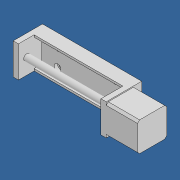
# Autodesk Inventor part: Linear_Unit_A
Saved by Autodesk Inventor 2020 (Build 240168000, 168)
## iProperties
Created: 2021-07-13
Part Number: Linear_Unit_A
Material: 一般
Document SubType Name: Modeling
Designer: ken113
Density: 1 g/cm^3
Appearance: 既定
Author: ken113
Autodesk Inventor part; units mm, degrees
ref_plane "YZ Plane" through (0, 0, 0) normal (1, 0, 0) x (0, 1, 0)
ref_plane "XZ Plane" through (0, 0, 0) normal (0, 1, 0) x (-1, 0, 0)
ref_plane "XY Plane" through (0, 0, 0) normal (0, 0, 1) x (1, 0, 0)
sketch "スケッチ1" plane through (0, 0, 0) normal (0, 0, 1) x (1, 0, 0)
  line L0 (62.5, -15) -> (-62.5, -15)
  line L1 (-62.5, -15) -> (-62.5, 15)
  line L2 (-62.5, 15) -> (62.5, 15)
  line L3 (62.5, 15) -> (62.5, -15)
  line L4 (62.5, -15) -> (-62.5, 15) construction
  line L5 (-62.5, -15) -> (62.5, 15) construction
  point P0 (0, 0)
  dimension "d0" = 30
  dimension "d1" = 125
  constraints: 12 end point, 2 midpoint, 2 parallel, 1 horizontal, 1 perpendicular
  measures "d0" distance of L0.end L1.end
  measures "d1" distance of L1.end L2.end
extrude "押し出し1" add sketch "スケッチ1" along normal blind 34
sketch "スケッチ2" plane through (-62.5, 15, 0) normal (0, 1, 0) x (1, 0, 0)
  line L0 (125, 0) -> (95, 0)
  line L1 (95, 0) -> (95, -6)
  line L2 (95, -6) -> (125, -6)
  line L3 (125, -6) -> (125, 0)
  point P0 (62.5, 0)
  dimension "d4" = 30
  dimension "d5" = 6
  constraints: 8 end point, 2 parallel, 1 horizontal, 1 perpendicular
  measures "d4" distance of L1.end L2.end
  measures "d5" distance of L0.end L1.end
extrude "押し出し2" cut sketch "スケッチ2" against normal blind 34
sketch "スケッチ3" plane through (-62.5, 15, 34) normal (0, 1, 0) x (1, 0, 0)
  line L0 (0, 0) -> (125, 0) projected
  line L1 (90, 0) -> (5, 0)
  line L2 (5, 0) -> (5, 21)
  line L3 (5, 21) -> (90, 21)
  line L4 (90, 21) -> (90, 0)
  line L5 (0, 34) -> (0, 0) projected
  line L6 (95, 28) -> (95, 34) projected
  line L7 (95, 34) -> (0, 34) projected
  point P0 (62.5, 34)
  point P1 (5, 0)
  dimension "d8" = 5
  dimension "d9" = 5
  dimension "d10" = 13
  constraints: 8 end point, 2 parallel, 1 horizontal, 1 perpendicular, 1 point on line
  measures "d8" distance between parallel lines of L5 L2
  measures "d9" distance between parallel lines of L4 L6
  measures "d10" distance between parallel lines of L3 L7
extrude "押し出し3" cut sketch "スケッチ3" against normal blind 34
sketch "スケッチ4" plane through (-62.5, 15, 34) normal (0, 1, 0) x (1, 0, 0)
  line L0 (90, 21) -> (90, 0) projected
  line L1 (125, 0) -> (90, 0) projected
  line L2 (125, 28) -> (125, 0) projected
  line L3 (125, 28) -> (95, 28) projected
  line L4 (95, 28) -> (95, 34) projected
  line L5 (95, 34) -> (0, 34) projected
  line L6 (0, 34) -> (0, 0) projected
  line L7 (5, 0) -> (0, 0) projected
  line L8 (5, 0) -> (5, 21) projected
  line L9 (5, 21) -> (90, 21) projected
  line L10 (5, 0) -> (5, 21) projected
  line L11 (5, 0) -> (0, 0)
  line L12 (0, 0) -> (0, 6)
  line L13 (0, 6) -> (5, 6)
  line L14 (5, 6) -> (5, 0)
  point P0 (62.5, 34)
  point P1 (5, 6)
  dimension "d13" = 28
  constraints: 8 end point, 2 parallel, 1 horizontal, 1 perpendicular, 1 point on line
  measures "d13" distance between parallel lines of L13 L5
extrude "押し出し4" cut sketch "スケッチ4" against normal blind 34 contours L8 L7 L6 L13
sketch "スケッチ5" plane through (0, 0, 0) normal (0, 0, -1) x (-1, 0, 0)
  line L0 (-12.5, 8.5) -> (42.5, 8.5)
  line L1 (42.5, 8.5) -> (42.5, -8.5)
  line L2 (42.5, -8.5) -> (-12.5, -8.5)
  line L3 (-12.5, -8.5) -> (-12.5, 8.5)
  line L4 (-32.5, 15) -> (-32.5, -15) projected
  line L5 (62.5, 15) -> (62.5, -15) projected
  point P0 (0, 0)
  dimension "d17" = 20
  dimension "d18" = 55
  dimension "d26" = 17
  dimension "d27" = 8.5
  constraints: 8 end point, 2 parallel, 1 horizontal, 1 perpendicular
  measures "d17" distance between parallel lines of L5 L1
  measures "d18" distance of L0.start L0.end
  measures "d26" distance of L0.end L1.end
  measures "d27" distance from line of L0 point (0, 0)
hole "穴1" at (12.5, 8.5, 0) at (12.5, -8.5, 0) at (-42.5, -8.5, 0) at (-42.5, 8.5, 0) direction (0, 0, 1) diameter 3.3 depth 23
sketch "スケッチ6" plane through (-57.5, 15, 13) normal (0, 0, 1) x (1, 0, 0)
  line L0 (85, -2) -> (0, -2)
  line L1 (0, -2) -> (0, -28)
  line L2 (0, -28) -> (85, -28)
  line L3 (85, -28) -> (85, -2)
  line L4 (0, 0) -> (85, 0) projected
  line L5 (85, -30) -> (0, -30) projected
  point P0 (57.5, -15)
  dimension "d28" = 2
  dimension "d29" = 2
  constraints: 8 end point, 2 parallel, 2 vertical alignment, 1 horizontal, 1 perpendicular
  measures "d28" distance between parallel lines of L0 L4
  measures "d29" distance between parallel lines of L5 L2
extrude "押し出し5" cut sketch "スケッチ6" against normal blind 7.5
sketch "スケッチ7" plane through (-57.5, 15, 5.5) normal (0, 0, 1) x (1, 0, 0)
  circle A0 centre (15, -23.5) radius 1.65 projected
  circle A1 centre (70, -6.5) radius 1.65 projected
  circle A2 centre (70, -23.5) radius 1.65 projected
  circle A3 centre (15, -6.5) radius 1.65 projected
  line L0 (85, -2) -> (85, -28) projected
  line L1 (0, -2) -> (85, -2) projected
  line L2 (0, -28) -> (0, -2) projected
  line L3 (85, -28) -> (0, -28) projected
  point P0 (57.5, -15)
hole "穴2" at (12.5, 8.5, 5.5) at (-42.5, 8.5, 5.5) at (-42.5, -8.5, 5.5) at (12.5, -8.5, 5.5) direction (0, 0, -1) diameter 3.3 depth 23 counterbore diameter 6.5 counterbore depth 3
sketch "スケッチ8" plane through (0, 0, 34) normal (0, 0, 1) x (1, 0, 0)
  line L0 (62.5, 15) -> (32.5, 15) projected
  line L1 (62.5, -15) -> (62.5, 15) projected
  line L2 (32.5, 15) -> (62.5, 15)
  line L3 (62.5, 15) -> (62.5, 14)
  line L4 (62.5, 14) -> (32.5, 14)
  line L5 (32.5, 14) -> (32.5, 15)
  line L6 (62.5, -15) -> (32.5, -15)
  line L7 (32.5, -15) -> (32.5, -14)
  line L8 (32.5, -14) -> (62.5, -14)
  line L9 (62.5, -14) -> (62.5, -15)
  point P0 (0, 0)
  dimension "d39" = 28
  dimension "d40" = 14
  constraints: 16 end point, 4 parallel, 2 horizontal, 2 perpendicular, 2 point on line
  measures "d39" distance between parallel lines of L8 L4
  measures "d40" distance from line of point (0, 0) L8
extrude "押し出し6" cut sketch "スケッチ8" against normal through all
chamfer "面取り1" distance 2 angle 45 4 edges at (47.5, 14, 34) (47.5, -14, 34) (47.5, 14, 6) (47.5, -14, 6)
sketch "スケッチ9" plane through (-62.5, -15, 0) normal (-1, 0, 0) x (0, 0, 1)
  line L0 (28, 0) -> (28, 30) projected
  line L1 (0, 30) -> (28, 30) projected
  line L2 (0, 30) -> (0, 0) projected
  line L3 (0, 0) -> (28, 0) projected
  circle A0 centre (20, 15) radius 3
  point P0 (0, 15)
  dimension "d46" = 20
  dimension "d47" = 6
  constraints: 1 centre point, 1 coincident
  measures "d46" distance from line of point (20, 15) L2
  measures "d47" diameter of A0
extrude "押し出し7" add sketch "スケッチ9" against normal up to surface (90 mm away) contours A0
